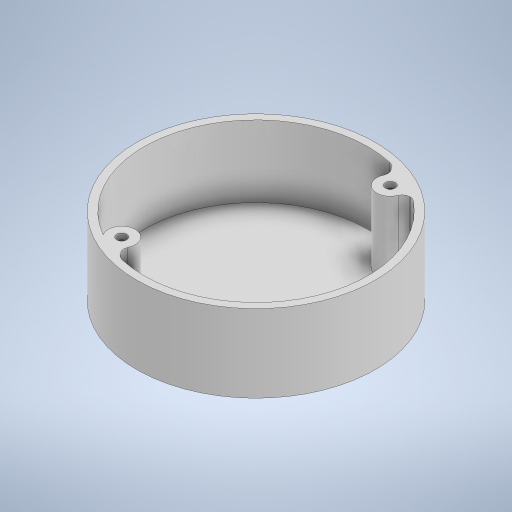
# Autodesk Inventor part: C0-0-01-ODriveCover
Saved by Autodesk Inventor 2023 (Build 270158000, 158)
## iProperties
Created: 2023-11-01
Part Number: C0-0-01-ODriveCover
Material: Generic
Document SubType Name: Modeling
Designer: thesl
Density: 1 g/cm^3
Appearance: Default
Author: thesl
Autodesk Inventor part; units mm, degrees
ref_plane "YZ Plane" through (0, 0, 0) normal (1, 0, 0) x (0, 1, 0)
ref_plane "XZ Plane" through (0, 0, 0) normal (0, 1, 0) x (-1, 0, 0)
ref_plane "XY Plane" through (0, 0, 0) normal (0, 0, 1) x (1, 0, 0)
sketch "Sketch1" plane through (0, 0, 0) normal (0, 1, 0) x (-1, 0, 0)
  circle A0 centre (0, 0) radius 50.8
  dimension "d0" = 101.6
  constraints: 1 centre point, 1 coincident
  measures "d0" diameter of A0
extrude "Extrusion1" add sketch "Sketch1" along normal blind 2.54
sketch "Sketch2" plane through (0, 2.54, 0) normal (0, 1, 0) x (1, 0, 0)
  circle A0 centre (0, 0) radius 47.625
  circle A1 centre (0, 0) radius 50.8
  dimension "d3" = 95.25
  dimension "d4" = 101.6
  constraints: 2 centre point, 1 coincident
  measures "d3" diameter of A0
  measures "d4" diameter of A1
extrude "Extrusion2" add sketch "Sketch2" along normal blind 30.48
sketch "Sketch3" plane through (0, 2.54, 0) normal (0, 1, 0) x (1, 0, 0)
  line L0 (0, 0) -> (0, 38.1)
  line L1 (0, 0) -> (0, -38.1)
  line L2 (0, -38.1) -> (-19.05, -38.1)
  line L3 (0, 38.1) -> (19.05, 38.1)
  circle A0 centre (19.05, 38.1) radius 5.715
  circle A1 centre (-19.05, -38.1) radius 5.715
  dimension "d9" = 38.1
  dimension "d10" = 19.05
  dimension "d11" = 11.43
  dimension "d12" = 11.43
  constraints: 8 end point, 2 centre point, 2 coincident, 2 vertical, 1 horizontal, 1 perpendicular
  measures "d9" distance of L0.start L1.end
  measures "d10" distance of L0.end L3.end
  measures "d11" diameter of A0
  measures "d12" diameter of A1
extrude "Extrusion3" add sketch "Sketch3" along normal blind 30.48
sketch "Sketch4" plane through (0, 2.54, 0) normal (0, 1, 0) x (1, 0, 0)
  arc A0 (18.6915, 43.8037) -> (23.8281, 41.2355) centre (19.05, 38.1) ccw projected
  line L0 (19.05, 38.1) -> (11.4832, 46.2199)
  arc A1 (-18.6915, -43.8037) -> (23.8281, 41.2355) centre (0, 0) ccw projected
  line L1 (19.05, 38.1) -> (29.6369, 38.1)
  line L2 (29.6369, 38.1) -> (22.8712, 45.3602)
  circle A2 centre (0, 0) radius 50.8 projected
  arc A3 (-18.6915, -43.8037) -> (-23.8281, -41.2355) centre (-19.05, -38.1) ccw projected
  line L3 (-19.05, -38.1) -> (-28.575, -38.1)
  line L4 (-19.05, -38.1) -> (-11.4832, -46.2199)
  line L5 (-21.0799, -46.2199) -> (-28.575, -38.1)
  line L6 (11.4832, 46.2199) -> (21.0799, 46.2199)
  line L7 (21.0799, 46.2199) -> (22.8712, 45.3602)
  line L8 (-11.4832, -46.2199) -> (-21.0799, -46.2199)
  line L9 (-21.0799, -46.2199) -> (-28.575, -38.1)
  point P0 (-15.1538, -42.281)
  point P1 (-24.765, -38.1)
  constraints: 20 end point, 6 point on circle, 4 horizontal, 1 collinear, 1 parallel
extrude "Extrusion4" add sketch "Sketch4" along normal blind 30.48 contours L0 L6 L7 L2 L1 A1 A0 | A0 A1 L1 | A1 A3 L4 | L4 L3 A3
fillet "Fillet1" radius 3.175 6 edges at (24.765, 17.78, -38.1) (28.575, 17.78, -38.1) (11.4832, 17.78, -46.2199) (15.1538, 17.78, -42.281) (-11.4832, 17.78, 46.2199) (-15.1538, 17.78, 42.281)
sketch "Sketch5" plane through (0, 33.02, 0) normal (0, 1, 0) x (1, 0, 0)
  arc A0 (13.9175, 40.6138) -> (24.3881, 36.0589) centre (19.05, 38.1) ccw projected
  line L0 (19.05, 32.385) -> (19.05, 38.1)
  arc A1 (-13.9175, -40.6138) -> (-23.8281, -41.2355) centre (-19.05, -38.1) ccw projected
  line L1 (-19.05, -32.385) -> (-19.05, -38.1)
  point P0 (0, 0)
  point P1 (-22.4437, -36.3682)
  constraints: 4 end point, 2 point on circle, 2 vertical
hole "Hole1" at (19.05, 33.02, -38.1) at (-19.05, 33.02, 38.1) direction (0, -1, 0) diameter 4.2926 end through all clearance for "Socket Head Cap Screw" size "M4" standard "Ansi Metric M Profile"
sketch "Sketch6" plane through (0, 0, 0) normal (0, -1, 0) x (1, 0, 0)
  point P0 (0, 0)
sketch "Sketch7" plane through (0, 0, 0) normal (0, -1, 0) x (1, 0, 0)
  circle A0 centre (19.05, -38.1) radius 2.1463 projected
  circle A1 centre (19.05, -38.1) radius 3.8076
  circle A2 centre (-19.05, 38.1) radius 2.1463 projected
  circle A3 centre (-19.05, 38.1) radius 3.81
  point P0 (0, 0)
  dimension "d25" = 7.62
  constraints: 2 centre point, 2 coincident
  measures "d25" diameter of A3
extrude "Extrusion5" cut sketch "Sketch7" against normal blind 30.48 contours A0 | A1 | A2 | A3
fillet "Fillet2" radius 3.175 1 edges at (15.2424, 30.48, -38.1)
fillet "Fillet3" radius 3.175 1 edges at (-22.86, 30.48, 38.1)
body "Solid1"
